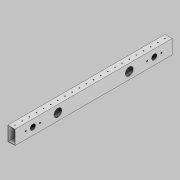
# Autodesk Inventor part: VerseFrame 22in for Ball Suck
Saved by Autodesk Inventor 2021.2 (Build 252289000, 289)
## iProperties
Created: 2020-01-13
Part Number: VerseFrame 22in for Ball Suck
Material: Generic
Document SubType Name: Modeling
Designer: aidan
Density: 1 g/cm^3
Appearance: Default
Author: aidan
Autodesk Inventor part; units mm, degrees
ref_plane "YZ Plane" through (0, 0, 0) normal (1, 0, 0) x (0, 1, 0)
ref_plane "XZ Plane" through (0, 0, 0) normal (0, 1, 0) x (-1, 0, 0)
ref_plane "XY Plane" through (0, 0, 0) normal (0, 0, 1) x (1, 0, 0)
sketch "Sketch1" plane through (0, 0, 0) normal (0, 0, 1) x (1, 0, 0)
  line L0 (-12.1708, 16.0073) -> (13.2292, 16.0073)
  line L1 (13.2292, 16.0073) -> (13.2292, -34.7927)
  line L2 (13.2292, -34.7927) -> (-12.1708, -34.7927)
  line L3 (-12.1708, -34.7927) -> (-12.1708, 16.0073)
  line L4 (11.9592, 14.7373) -> (-10.9008, 14.7373)
  line L5 (-10.9008, 14.7373) -> (-10.9008, -33.5227)
  line L6 (-10.9008, -33.5227) -> (11.9592, -33.5227)
  line L7 (11.9592, -33.5227) -> (11.9592, 14.7373)
  point P0 (0, 0)
  dimension "d0" = 25.4
  dimension "d1" = 50.8
  dimension "d2" = 1.27
  constraints: 16 end point, 4 parallel, 2 perpendicular, 1 horizontal, 3 other
  measures "d0" distance of L0.start L0.end
  measures "d1" distance of L0.end L1.end
  measures "d2" distance between parallel lines of L0 L4
extrude "Extrusion1" add sketch "Sketch1" along normal blind 558.8
sketch "Sketch2" plane through (-12.1708, 16.0073, 0) normal (0, 1, 0) x (1, 0, 0)
  circle A0 centre (12.7, -12.7) radius 1.7272
  line L0 (25.4, 0) -> (0, 0) projected
  line L1 (0, 0) -> (0, -558.8) projected
  point P0 (12.1708, 0)
  dimension "d5" = 3.4544
  dimension "d6" = 12.7
  dimension "d7" = 12.7
  constraints: 1 centre point
  measures "d5" diameter of A0
  measures "d6" distance from line of L0 A0.centre
  measures "d7" distance from line of L1 A0.centre
extrude "Extrusion2" cut sketch "Sketch2" against normal through all
pattern_linear "Rectangular Pattern1" count 22 spacing 25.4 along (0, 0, 1) of "Extrusion2"
sketch "Sketch4" plane through (13.2292, -34.7927, 0) normal (1, 0, 0) x (0, 0, -1)
  circle A0 centre (-406.4, 25.4) radius 14.2875
  circle A1 centre (-152.4, 25.4) radius 14.2875
  circle A2 centre (-495.3, 25.4) radius 9.525
  circle A3 centre (-63.5, 25.4) radius 9.525
  line L0 (-495.3, 25.4) -> (-63.5, 25.4) construction
  line L1 (0, 50.8) -> (-558.8, 50.8) projected
  line L2 (0, 0) -> (-558.8, 0) projected
  line L3 (-279.4, 0) -> (-279.4, 50.8) construction
  line L4 (0, 0) -> (0, 50.8) projected
  line L5 (-558.8, 0) -> (-558.8, 50.8) projected
  point P0 (0, 34.7927)
  dimension "d15" = 28.575
  dimension "d16" = 25.4
  dimension "d17" = 254
  dimension "d18" = 279.4
  dimension "d19" = 127
  dimension "d20" = 88.9
  dimension "d22" = 88.9
  dimension "d23" = 19.05
  dimension "d24" = 558.8
  constraints: 4 centre point, 4 end point, 2 equal radius, 2 midpoint, 2 point on line, 1 horizontal, 1 vertical
  measures "d15" diameter of A0
  measures "d16" distance between parallel lines of L1 L0
  measures "d17" distance of A1.centre A0.centre
  measures "d18" distance between parallel lines of L4 L3
  measures "d19" distance from line of L3 A1.centre
  measures "d20" distance of A0.centre L0.start
  measures "d22" distance of L0.end A1.centre
  measures "d23" diameter of A3
  measures "d24" distance between parallel lines of L4 L5
extrude "Extrusion3" cut sketch "Sketch4" against normal through all contours A0 | A1 | A2 | A3
sketch "Sketch5" plane through (13.2292, -34.7927, 0) normal (1, 0, 0) x (0, 0, -1)
  circle A0 centre (-495.3, 25.4) radius 9.525 projected
  circle A1 centre (-63.5, 25.4) radius 9.525 projected
  circle A2 centre (-495.3, 25.4) radius 25.4 construction
  circle A3 centre (-63.5, 25.4) radius 25.4 construction
  circle A4 centre (-495.3, 25.4) radius 9.525 projected
  line L0 (-495.3, 25.4) -> (-63.5, 25.4) construction
  circle A5 centre (-469.9, 25.4) radius 2.5797
  circle A6 centre (-520.7, 25.4) radius 2.5797
  circle A7 centre (-88.9, 25.4) radius 2.5797
  circle A8 centre (-38.1, 25.4) radius 2.5797
  point P0 (0, 34.7927)
  dimension "d27" = 50.8
  dimension "d28" = 5.1594
  constraints: 6 centre point, 4 equal radius, 4 point on circle, 4 point on line, 2 coincident, 2 end point, 1 horizontal
  measures "d27" diameter of A2
  measures "d28" diameter of A6
extrude "Extrusion4" cut sketch "Sketch5" against normal through all contours A5 | A6 | A7 | A8
equation "\"d3\" = d13"
equation "\"d13\" = 558.8"
body "Solid1"
